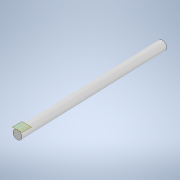
# Autodesk Inventor part: trail 15
Saved by Autodesk Inventor 2020.2 (Build 242310000, 310)
## iProperties
Created: 2020-03-01
Part Number: trail 15
Material: Generic
Document SubType Name: Modeling
Designer: lenovo
Density: 1 g/cm^3
Appearance: Default
Author: lenovo
Autodesk Inventor part; units mm, degrees
ref_plane "YZ Plane" through (0, 0, 0) normal (1, 0, 0) x (0, 1, 0)
ref_plane "XZ Plane" through (0, 0, 0) normal (0, 1, 0) x (-1, 0, 0)
ref_plane "XY Plane" through (0, 0, 0) normal (0, 0, 1) x (1, 0, 0)
ref_plane "Work Plane1" through (164.2028, -83.8114, 405.2203) normal (0, -1, 0) x (0, 0, 1)
sketch "Sketch1" plane through (164.2028, -83.8114, 405.2203) normal (0, -1, 0) x (0, 0, 1)
  line L0 (10, -10) -> (-334.7898, 2.0403)
  line L1 (-334.7898, 2.0403) -> (-334.0918, 22.0281)
  line L2 (-334.0918, 22.0281) -> (10.698, 9.9878)
  line L3 (10.698, 9.9878) -> (10, -10)
  line L4 (10, -10) -> (355, -10) construction
  point P0 (-405.2203, 164.2028)
  dimension "d0" = 345
  dimension "d1" = 178
  dimension "d2" = 20
  constraints: 10 end point, 2 parallel, 1 equal length, 1 horizontal, 1 perpendicular
  measures "d0" distance of L0.start L0.end
  measures "d1" angle of L4 L0
  measures "d2" distance of L0.end L1.end
extrude "Extrusion1" add sketch "Sketch1" along normal blind 20
sketch "Sketch2" plane through (154.215, -103.8114, 415.9183) normal (0.0348995, 0, 0.9993908) x (0.9993908, 0, -0.0348995)
  circle A0 centre (10, 10) radius 10
  line L0 (20, 20) -> (0, 20) projected
  point P0 (-139.6057, 103.8114)
  constraints: 1 centre point, 1 tangent
extrude "Extrusion2" cut sketch "Sketch2" against normal blind 345 keep common part
body "Solid1"
